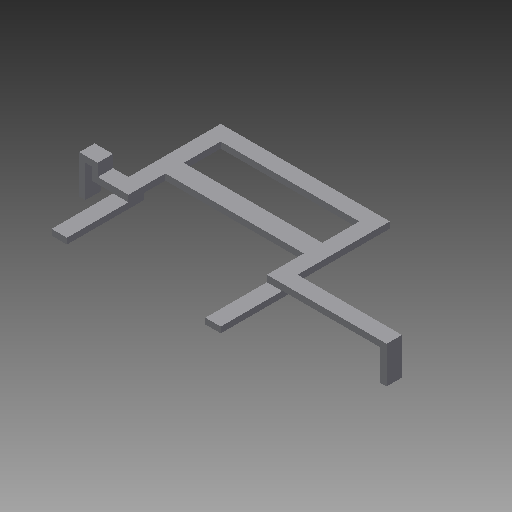
# Autodesk Inventor part: Steunbalk boven bocht
Saved by Autodesk Inventor 2018.3 (Build 223284000, 284)
## iProperties
Created: 2020-11-17
Part Number: Steunbalk boven bocht
Material: Generic
Document SubType Name: Modeling
Designer: daanv
Density: 1 g/cm^3
Appearance: Default
Author: daanv
Autodesk Inventor part; units mm, degrees
ref_plane "YZ Plane" through (0, 0, 0) normal (1, 0, 0) x (0, 1, 0)
ref_plane "XZ Plane" through (0, 0, 0) normal (0, 1, 0) x (-1, 0, 0)
ref_plane "XY Plane" through (0, 0, 0) normal (0, 0, 1) x (1, 0, 0)
sketch "Sketch1" plane through (0, 0, 0) normal (0, 0, 1) x (1, 0, 0)
  line L0 (0, 0) -> (2, 0)
  line L1 (2, 0) -> (2, 12.5)
  line L2 (2, 12.5) -> (0, 12.5)
  line L3 (0, 12.5) -> (0, 0)
  line L4 (2, 12.5) -> (6, 12.5)
  line L5 (6, 12.5) -> (6, 10.5)
  line L6 (6, 10.5) -> (2, 10.5)
  line L7 (2, 10.5) -> (2, 12.5)
  line L8 (6, 10.5) -> (4, 10.5)
  line L9 (4, 10.5) -> (4, 6.5)
  line L10 (4, 6.5) -> (6, 6.5)
  line L11 (6, 6.5) -> (6, 10.5)
  dimension "d0" = 2
  dimension "d1" = 12.5
  dimension "d2" = 4
  dimension "d3" = 2
  dimension "d4" = 2
  dimension "d5" = 4
  constraints: 24 end point, 6 parallel, 3 horizontal, 3 perpendicular
  measures "d0" distance of L2.end L1.end
  measures "d1" distance of L1.end L0.end
  measures "d2" distance of L5.end L6.end
  measures "d3" distance of L4.end L5.end
  measures "d4" distance of L10.end L9.end
  measures "d5" distance of L9.end L8.end
extrude "Extrusion1" add sketch "Sketch1" along normal blind 5
sketch "Sketch2" plane through (6, 6.5, 0) normal (1, 0, 0) x (0, 0, -1)
  line L0 (-5, 4) -> (-5, 0) projected
  line L1 (0, 0) -> (0, 4) projected
  line L2 (-5, 0) -> (0, 0)
  line L3 (0, 0) -> (0, 2)
  line L4 (0, 2) -> (-5, 2)
  line L5 (-5, 2) -> (-5, 0)
  point P0 (0, -6.5)
  dimension "d8" = 2
  constraints: 8 end point, 2 parallel, 1 horizontal, 1 midpoint, 1 perpendicular
  measures "d8" distance of L3.end L2.end
extrude "Extrusion2" add sketch "Sketch2" along normal blind 10
sketch "Sketch3" plane through (0, 0, 0) normal (0, 0, -1) x (-1, 0, 0)
  line L0 (-16, 6.5) -> (-4, 6.5) projected
  line L1 (-16, 8.5) -> (-16, 6.5) projected
  line L2 (-16, 8.5) -> (-11, 8.5)
  line L3 (-11, 8.5) -> (-11, 6.5)
  line L4 (-11, 6.5) -> (-16, 6.5)
  line L5 (-16, 6.5) -> (-16, 8.5)
  constraints: 8 end point, 2 parallel, 1 horizontal, 1 perpendicular, 1 point on line
extrude "Extrusion3" add sketch "Sketch3" along normal blind 30
sketch "Sketch4" plane through (16, 6.5, 0) normal (1, 0, 0) x (0, 0, -1)
  line L0 (-5, 0) -> (30, 0) projected
  line L1 (30, 0) -> (30, 2) projected
  line L2 (30, 2) -> (25, 2)
  line L3 (25, 2) -> (25, 0)
  line L4 (25, 0) -> (30, 0)
  line L5 (30, 0) -> (30, 2)
  point P0 (0, -6.5)
  dimension "d13" = 5
  constraints: 8 end point, 2 parallel, 1 horizontal, 1 perpendicular, 1 point on line
  measures "d13" distance of L4.end L3.end
extrude "Extrusion4" add sketch "Sketch4" along normal blind 50
sketch "Sketch5" plane through (16, 6.5, -25) normal (0, 0, 1) x (1, 0, 0)
  line L0 (-5, 0) -> (50, 0) projected
  line L1 (50, 2) -> (45, 2)
  line L2 (45, 2) -> (45, 0)
  line L3 (45, 0) -> (50, 0)
  line L4 (50, 0) -> (50, 2)
  point P0 (-16, -6.5)
  dimension "d16" = 5
  constraints: 8 end point, 2 parallel, 1 horizontal, 1 perpendicular, 1 point on line
  measures "d16" distance of L3.end L2.end
extrude "Extrusion5" add sketch "Sketch5" along normal blind 30
sketch "Sketch6" plane through (66, 6.5, 0) normal (1, 0, 0) x (0, 0, -1)
  line L0 (0, 0) -> (-5, 0) projected
  line L1 (-5, 2) -> (0, 2)
  line L2 (0, 2) -> (0, 0)
  line L3 (0, 0) -> (-5, 0)
  line L4 (-5, 0) -> (-5, 2)
  point P0 (0, -6.5)
  constraints: 8 end point, 2 parallel, 1 horizontal, 1 perpendicular
extrude "Extrusion6" add sketch "Sketch6" along normal blind 29.93
sketch "Sketch7" plane through (95.93, 6.5, 0) normal (1, 0, 0) x (0, 0, -1)
  line L0 (0, 0) -> (0, 2) projected
  line L1 (0, 2) -> (-5, 2) projected
  line L2 (-5, 2) -> (-5, 0) projected
  line L3 (-5, 0) -> (0, 0) projected
  point P0 (0, -6.5)
extrude "Extrusion7" add sketch "Sketch7" along normal blind 4
sketch "Sketch8" plane through (4, 6.5, 0) normal (0, -1, 0) x (1, 0, 0)
  line L0 (62, 0) -> (95.93, 0) projected
  line L1 (57, 5) -> (95.93, 5) projected
  line L2 (95.93, 5) -> (93.93, 5)
  line L3 (93.93, 5) -> (93.93, 0)
  line L4 (93.93, 0) -> (95.93, 0)
  line L5 (95.93, 0) -> (95.93, 5)
  point P0 (-4, 0)
  dimension "d23" = 2
  constraints: 8 end point, 2 parallel, 1 horizontal, 1 perpendicular, 1 point on line
  measures "d23" distance of L4.end L3.end
extrude "Extrusion8" add sketch "Sketch8" along normal blind 10
sketch "Sketch9" plane through (4, 6.5, 0) normal (0, -1, 0) x (1, 0, 0)
  line L0 (57, 5) -> (95.93, 5) projected
  line L1 (62, 0) -> (95.93, 0) projected
  line L2 (57, 5) -> (62, 5)
  line L3 (62, 5) -> (62, 0)
  line L4 (62, 0) -> (57, 0)
  line L5 (57, 0) -> (57, 5)
  line L6 (12, 5) -> (7, 5)
  line L7 (7, 5) -> (7, 0)
  line L8 (7, 0) -> (12, 0)
  line L9 (12, 0) -> (12, 5)
  line L10 (7, 5) -> (12, 5)
  line L11 (12, 5) -> (12, 0)
  line L12 (12, 0) -> (7, 0)
  line L13 (7, 0) -> (7, 5)
  line L14 (57, 5) -> (62, 5)
  line L15 (62, 5) -> (62, 0)
  line L16 (62, 0) -> (57, 0)
  line L17 (57, 0) -> (57, 5)
  point P0 (-4, 0)
  constraints: 32 end point, 8 parallel, 4 horizontal, 4 perpendicular
extrude "Extrusion9" add sketch "Sketch9" along normal blind 2
sketch "Sketch10" plane through (0, 0, 5) normal (0, 0, 1) x (1, 0, 0)
  line L0 (16, 8.5) -> (16, 4.5) projected
  line L1 (11, 4.5) -> (16, 4.5)
  line L2 (16, 4.5) -> (16, 6.4)
  line L3 (16, 6.4) -> (11, 6.4)
  line L4 (11, 6.4) -> (11, 4.5)
  dimension "d28" = 1.9
  constraints: 8 end point, 2 parallel, 1 horizontal, 1 perpendicular, 1 point on line
  measures "d28" distance of L2.end L1.end
extrude "Extrusion10" add sketch "Sketch10" along normal blind 20
sketch "Sketch11" plane through (16, 6.5, 5) normal (0, 0, 1) x (1, 0, 0)
  line L0 (50, 0) -> (50, -2) projected
  line L1 (45, -2) -> (50, -2)
  line L2 (50, -2) -> (50, -0.1)
  line L3 (50, -0.1) -> (45, -0.1)
  line L4 (45, -0.1) -> (45, -2)
  point P0 (-16, -6.5)
  dimension "d31" = 1.9
  constraints: 8 end point, 2 parallel, 1 horizontal, 1 perpendicular, 1 point on line
  measures "d31" distance of L2.end L1.end
extrude "Extrusion11" add sketch "Sketch11" along normal blind 20
sketch "Sketch12" plane through (61, 6.5, -25) normal (-1, 0, 0) x (0, 0, 1)
  line L0 (0, 0) -> (25, 0) projected
  line L1 (30, 2) -> (30, -0.1) projected
  line L2 (0, 2) -> (30, 2) projected
  line L3 (12, 2) -> (18, 2)
  line L4 (18, 2) -> (18, 0)
  line L5 (18, 0) -> (12, 0)
  line L6 (12, 0) -> (12, 2)
  point P0 (25, -6.5)
  dimension "d34" = 6
  dimension "d35" = 12
  constraints: 8 end point, 2 parallel, 2 point on line, 1 horizontal, 1 perpendicular
  measures "d34" distance of L4.end L5.end
  measures "d35" distance between parallel lines of L1 L4
extrude "Extrusion12" add sketch "Sketch12" along normal up to next
body "Solid1"
